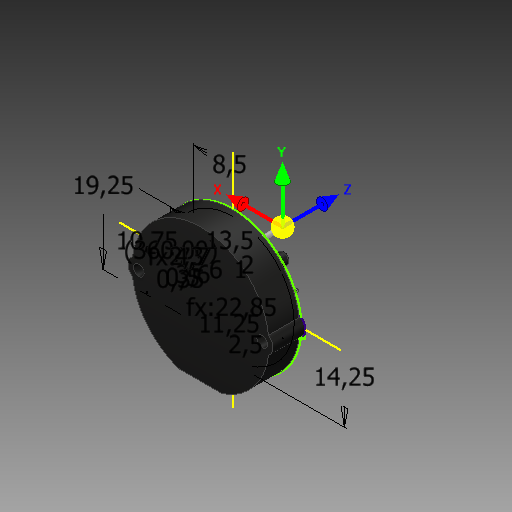
# Autodesk Inventor part: VID26
Saved by Autodesk Inventor 2019 (Build 230136000, 136)
## iProperties
Created: 2018-04-28
Part Number: VID26
Material: PBT Plastic
Document SubType Name: Modeling
Designer: Fierl
Density: 1.31 g/cm^3
Appearance: Smooth - White
Mass: 6.22484 g
Surface Area: 22.8247 cm^2
Volume: 4.75179 cm^3
Author: Fierl
Autodesk Inventor part; units mm, degrees
ref_plane "YZ Plane" through (0, 0, 0) normal (1, 0, 0) x (0, 1, 0)
ref_plane "XZ Plane" through (0, 0, 0) normal (0, 1, 0) x (-1, 0, 0)
ref_plane "XY Plane" through (0, 0, 0) normal (0, 0, 1) x (1, 0, 0)
sketch "Sketch1" plane through (0, 0, 0) normal (0, 0, 1) x (1, 0, 0)
  line L0 (-24.6776, 0) -> (23.5544, 0) projected
  line L1 (0, -22.6406) -> (0, 25.7747) projected
  circle A0 centre (-13.5, 0) radius 1.15
  circle A1 centre (-13.5, 0) radius 2.35
  circle A2 centre (13.5, 0) radius 1.15
  circle A3 centre (13.5, 0) radius 2.35
  circle A4 centre (0, 6) radius 1
  circle A5 centre (0, 6) radius 0.5
  circle A6 centre (0, -10.75) radius 1.25
  circle A7 centre (-8.5, 8.5) radius 1.25
  circle A8 centre (8.5, 8.5) radius 1.25
  line L2 (-11.6, -3.6) -> (-11.25, -3.6)
  line L3 (-11.25, -3.6) -> (-11.25, -4.1)
  line L4 (-11.25, -4.1) -> (-11.6, -4.1)
  line L5 (-11.6, -4.1) -> (-11.6, -3.6)
  line L6 (11.25, -4.1) -> (11.25, -3.6)
  line L7 (11.25, -3.6) -> (11.6, -3.6)
  line L8 (11.6, -3.6) -> (11.6, -4.1)
  line L9 (11.6, -4.1) -> (11.25, -4.1)
  line L10 (-11.6, 3.6) -> (-11.6, 4.1)
  line L11 (-11.6, 4.1) -> (-11.25, 4.1)
  line L12 (-11.25, 4.1) -> (-11.25, 3.6)
  line L13 (-11.25, 3.6) -> (-11.6, 3.6)
  line L14 (11.25, 3.6) -> (11.25, 4.1)
  line L15 (11.25, 4.1) -> (11.6, 4.1)
  line L16 (11.6, 4.1) -> (11.6, 3.6)
  line L17 (11.6, 3.6) -> (11.25, 3.6)
  arc A9 (14.8788, 1.903) -> (4.6837, 14.25) centre (0, 0) ccw
  arc A10 (4.6837, 14.25) -> (-14.8788, 1.903) centre (0, 0) ccw
  arc A11 (4.6837, -14.25) -> (14.8788, -1.903) centre (0, 0) ccw
  circle A12 centre (5.4353, -14.25) radius 0.1148
  line L18 (-4.6837, -14.25) -> (4.6837, -14.25)
  arc A13 (14.8788, 1.903) -> (-14.8788, 1.903) centre (0, 0) ccw
  arc A14 (-14.8788, -1.903) -> (-14.5616, -3.6) centre (0, 0) ccw
  arc A15 (-14.5616, -3.6) -> (-4.6837, -14.25) centre (0, 0) ccw
  arc A16 (-14.5616, 3.6) -> (-14.8788, 1.903) centre (0, 0) ccw
  arc A17 (0, 15) -> (-14.5616, 3.6) centre (0, 0) ccw
  arc A18 (-14.5616, 3.6) -> (-14.8788, 1.903) centre (0, 0) ccw
  point P0 (-15.6415, -0.9678)
  point P1 (0, -15.6714)
  point P2 (15.1605, -1.6629)
  dimension "d2" = 2.3
  dimension "d3" = 4.7
  dimension "d4" = 13.5
  dimension "d7" = 360
  dimension "d9" = 2
  dimension "d10" = 1
  dimension "d11" = 6
  dimension "d12" = 2.5
  dimension "d13" = 10.75
  dimension "d14" = 19.25
  dimension "d16" = 8.5
  dimension "d17" = 0.35
  dimension "d18" = 0.5
  dimension "d19" = 11.25
  dimension "d20" = 3.6
  dimension "d23" = 22.85
  dimension "d26" = 7.7
  dimension "d48" = 14.25
  constraints: 34 end point, 25 point on circle, 19 centre point, 6 coincident, 6 point on line, 3 parallel, 2 equal radius, 2 horizontal, 1 perpendicular, 1 vertical, 34 other
  measures "d2" diameter of A0
  measures "d3" diameter of A1
  measures "d4" distance of point (0, 0) A0.centre
  measures "d9" diameter of A4
  measures "d10" diameter of A5
  measures "d11" distance of point (0, 0) A4.centre
  measures "d12" diameter of A6
  measures "d13" distance of point (0, 0) A6.centre
  measures "d14" vertical distance of A7.centre A6.centre
  measures "d16" distance from line of L1 A7.centre
  measures "d17" distance of L3.end L4.end
  measures "d18" distance of L2.end L3.end
  measures "d19" distance from line of L1 L3.end
  measures "d20" distance from line of L0 L2.end
  measures "d23" distance of L4.end L6.start
  measures "d26" distance of L4.end L10.start
  measures "d48" distance between parallel lines of L0 L18
extrude "Extrusion1" add sketch "Sketch1" along normal blind 7 contours A0 L0 A1 | L0 A1 A0 | A1 A10 L1 A4 L0 | L0 L1 A6 L18 A15 A14 A1 | L1 A4 A10 A9 A3 L0 | L0 A3 A11 L18 L1 A6 | A3 L0 A2 | L0 A2 A3 | A6 L1 | L1 A6 | A4 L1 A5 | L1 A5 A4 | A5 L1 | L1 A5 | A7 | A8 | L2 L3 L4 L5 | L6 L7 L8 L9 | L10 L11 L12 L13 | L14 L15 L16 L17
sketch "Sketch2" plane through (0, 0, 0) normal (0, 0, -1) x (-1, 0, 0)
  point P0 (0, 0)
extrude "Extrusion2" add sketch "Sketch1" against normal blind 3 contours A6 L1 | L1 A6 | A7 | A8
fillet "Fillet1" radius 0.5 3 edges at (7.25, 8.5, -3) (-1.25, -10.75, -3) (-9.75, 8.5, -3)
extrude "Extrusion3" add sketch "Sketch1" against normal blind 10.95 contours A5 L1 | L1 A5
extrude "Extrusion4" add sketch "Sketch1" against normal blind 2.3 contours A4 L1 A5 | L1 A5 A4
extrude "Extrusion5" add sketch "Sketch1" against normal blind 2.8 contours L2 L3 L4 L5 | L6 L7 L8 L9 | L10 L11 L12 L13 | L14 L15 L16 L17
extrude "Extrusion6" cut sketch "Sketch1" along normal blind 0.3 contours A1 A10 L1 A4 L0 | L0 L1 A6 L18 A15 A14 A1 | L1 A4 A10 A9 A3 L0 | L0 A3 A11 L18 L1 A6
equation "\"d23\" = 2 * d19 + d17"
equation "\"d26\" = 2 * d20 + d18"
body "Solid1"
